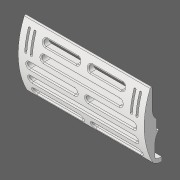
# Autodesk Inventor part: HandPlate
Saved by Autodesk Inventor 2020 (Build 240168000, 168)
## iProperties
Created: 2020-01-12
Part Number: HandPlate
Material: PLA Plastic (Black)
Document SubType Name: Modeling
Designer: Isaac Newcomb
Density: 1 g/cm^3
Appearance: 3D Printed - Black
Mass: 87.7555 g
Surface Area: 405.858 cm^2
Volume: 87.7555 cm^3
Author: Isaac Newcomb
Autodesk Inventor part; units mm, degrees
ref_plane "YZ Plane" through (0, 0, 0) normal (1, 0, 0) x (0, 1, 0)
ref_plane "XZ Plane" through (0, 0, 0) normal (0, 1, 0) x (-1, 0, 0)
ref_plane "XY Plane" through (0, 0, 0) normal (0, 0, 1) x (1, 0, 0)
sketch "Profile" plane through (0, 0, 0) normal (0, 0, 1) x (1, 0, 0)
  arc A0 (-13.7625, 56.5) -> (-16.6445, 57.0832) centre (-15.2625, 56.5) ccw
  line L0 (-7.7625, 0) -> (-7.7625, 15)
  arc A1 (-13.7625, 29.2829) -> (-7.7625, 15) centre (6.2375, 29.2829) ccw
  arc A2 (-16.6445, 57.0832) -> (-12.8608, -36.4892) centre (84.7024, 14.3185) ccw
  line L1 (0, 0) -> (-7.7625, 0)
  line L2 (-13.7625, 56.5) -> (-13.7625, 29.2829)
  line L3 (0, -41.5035) -> (0, -35.5035)
  line L4 (0, -35.5035) -> (-7.7625, -35.5035) construction
  arc A3 (-12.8608, -36.4892) -> (-12, -37.5035) centre (-10.2, -35.1035) ccw
  arc A4 (-9.8812, -31.3441) -> (-7.8643, -34.1785) centre (-6.8812, -31.3441) ccw
  arc A5 (-12, -37.5035) -> (0, -41.5035) centre (0, -21.5035) ccw
  line L5 (0, -41.5035) -> (-7.7625, -41.5035) construction
  arc A6 (-7.8643, -34.1785) -> (0, -35.5035) centre (0, -11.5035) ccw
  line L6 (-9.8812, -14.2829) -> (-9.8812, -31.3441)
  arc A7 (-3.8812, 0) -> (-9.8812, -14.2829) centre (10.1188, -14.2829) ccw
  dimension "height" = 56.5
  dimension "d3" = 1.5
  dimension "d5" = 15
  dimension "d100" = 110
  dimension "d114" = 20
  dimension "d115" = 7.7625
  dimension "d122" = 6
  dimension "d124" = 6
  dimension "d127" = 3
  dimension "d129" = 20
  dimension "d130" = 41.5035
  dimension "d131" = 12
  dimension "d133" = 20
  dimension "d134" = 6
  dimension "d135" = 3
  dimension "d136" = 10
  constraints: 17 point on circle, 14 end point, 10 tangent, 8 centre point, 4 vertical, 3 point on line, 2 midpoint, 2 perpendicular, 1 horizontal
  measures "height" vertical distance of A0.centre L1.start
  measures "d3" radius of A0
  measures "d5" distance of L0.start L0.end
  measures "d100" radius of A2
  measures "d114" radius of A1
  measures "d115" distance from line of L0 L1.start
  measures "d122" distance from line of L0 L2.start
  measures "d124" distance of L3.start L3.end
  measures "d127" radius of A3
  measures "d129" radius of A5
  measures "d130" distance of L1.start L3.start
  measures "d131" horizontal distance of L3.start A3.end
  measures "d133" radius of A7
  measures "d134" distance from line of A7.start L6
  measures "d135" radius of A4
  measures "d136" distance of A6.centre A5.centre
extrude "Extrusion" add sketch "Profile" along normal blind 180
sketch "Slot Sketch" plane through (0, 0, 0) normal (0, 1, 0) x (-1, 0, 0)
  line L0 (7.7625, 7.5) -> (10.7625, 9) construction
  line L1 (10.7625, 9) -> (10.7625, 3) construction
  line L2 (10.7625, 3) -> (7.7625, 4.5) construction
  line L3 (7.7625, 4.5) -> (7.7625, 7.5)
  line L4 (7.7625, 6) -> (11.2625, 6) construction
  line L5 (7.7625, 4.5) -> (7.7625, 3.941)
  line L6 (7.7625, 3.941) -> (11.2625, 2.191)
  line L7 (11.2625, 2.191) -> (11.2625, 9.809)
  line L8 (11.2625, 9.809) -> (7.7625, 8.059)
  line L9 (7.7625, 8.059) -> (7.7625, 7.5)
  line L10 (7.7625, 175.5) -> (10.7625, 177) construction
  line L11 (10.7625, 177) -> (10.7625, 171) construction
  line L12 (10.7625, 171) -> (7.7625, 172.5) construction
  line L13 (7.7625, 172.5) -> (7.7625, 175.5)
  line L14 (7.7625, 174) -> (11.2625, 174) construction
  line L15 (7.7625, 172.5) -> (7.7625, 171.941)
  line L16 (7.7625, 171.941) -> (11.2625, 170.191)
  line L17 (11.2625, 170.191) -> (11.2625, 177.809)
  line L18 (11.2625, 177.809) -> (7.7625, 176.059)
  line L19 (7.7625, 176.059) -> (7.7625, 175.5)
  line L20 (7.7625, 91.5) -> (10.7625, 93) construction
  line L21 (10.7625, 93) -> (10.7625, 87) construction
  line L22 (10.7625, 87) -> (7.7625, 88.5) construction
  line L23 (7.7625, 88.5) -> (7.7625, 91.5)
  line L24 (7.7625, 90) -> (11.2625, 90) construction
  line L25 (7.7625, 88.5) -> (7.7625, 87.941)
  line L26 (7.7625, 87.941) -> (11.2625, 86.191)
  line L27 (11.2625, 86.191) -> (11.2625, 93.809)
  line L28 (11.2625, 93.809) -> (7.7625, 92.059)
  line L29 (7.7625, 92.059) -> (7.7625, 91.5)
  point P0 (0, 0)
  point P1 (10.7625, 6)
  point P2 (10.7625, 174)
  point P3 (10.7625, 90)
  dimension "d14" = 0.5
  dimension "d15" = 0.5
  dimension "d16" = 3
  dimension "d17" = 6
  dimension "d18" = 3
  dimension "d19" = 7.7625
  dimension "d20" = 6
  dimension "d26" = 0.5
  dimension "d27" = 0.5
  dimension "d28" = 3
  dimension "d29" = 6
  dimension "d30" = 3
  dimension "d35" = 168
  dimension "d36" = 0.5
  dimension "d37" = 0.5
  dimension "d38" = 3
  dimension "d39" = 6
  dimension "d40" = 3
  dimension "d45" = 84
  constraints: 60 end point, 9 midpoint, 9 vertical, 6 parallel, 6 point on line, 5 collinear, 3 horizontal
  measures "d14" distance between parallel lines of L7 L1
  measures "d15" distance between parallel lines of L0 L8
  measures "d16" distance between parallel lines of L3 L1
  measures "d17" distance of L0.end L1.end
  measures "d18" distance of L2.end L0.start
  measures "d19" distance from line of point (0, 0) L3
  measures "d20" distance from line of point (0, 0) L4
  measures "d26" distance between parallel lines of L17 L11
  measures "d27" distance between parallel lines of L10 L18
  measures "d28" distance between parallel lines of L13 L11
  measures "d29" distance of L10.end L11.end
  measures "d30" distance of L12.end L10.start
  measures "d35" distance between parallel lines of L14 L4
  measures "d36" distance between parallel lines of L27 L21
  measures "d37" distance between parallel lines of L20 L28
  measures "d38" distance between parallel lines of L23 L21
  measures "d39" distance of L20.end L22.start
  measures "d40" distance of L22.end L23.end
  measures "d45" distance between parallel lines of L4 L24
extrude "Slots" cut sketch "Slot Sketch" along normal through all
sketch "Sketch3" plane through (0, 0, 0) normal (1, 0, 0) x (0, 1, 0)
  line L0 (50, 171) -> (20, 171)
  line L1 (20, 171) -> (20, 168)
  line L2 (20, 168) -> (50, 168)
  line L3 (50, 168) -> (50, 171)
  line L4 (50, 12) -> (20, 12)
  line L5 (20, 12) -> (20, 9)
  line L6 (20, 9) -> (50, 9)
  line L7 (50, 9) -> (50, 12)
  line L8 (35, 12) -> (35, 168) construction
  line L9 (20, 20) -> (50, 20)
  line L10 (50, 20) -> (50, 17)
  line L11 (50, 17) -> (20, 17)
  line L12 (20, 17) -> (20, 20)
  line L13 (20, 163) -> (50, 163)
  line L14 (50, 163) -> (50, 160)
  line L15 (50, 160) -> (20, 160)
  line L16 (20, 160) -> (20, 163)
  point P0 (0, 0)
  point P1 (35, 90)
  dimension "d48" = 90
  dimension "d50" = 20
  dimension "d51" = 30
  dimension "d52" = 3
  dimension "d53" = 12
  dimension "d56" = 5
  dimension "d57" = 5
  constraints: 34 end point, 8 parallel, 5 collinear, 4 horizontal, 4 perpendicular, 4 point on line, 3 midpoint
  measures "d48" vertical distance of point (0, 0) point (35, 90)
  measures "d50" distance from line of L5 point (0, 0)
  measures "d51" distance of L5.end L6.end
  measures "d52" distance of L6.end L4.start
  measures "d53" distance from line of point (0, 0) L4
  measures "d56" distance between parallel lines of L2 L13
  measures "d57" distance between parallel lines of L4 L11
extrude "Extrusion3" cut sketch "Sketch3" against normal through all
fillet "Fillet2" radius 1.5 16 edges at (-16.5561, 50, 12) (-18.3143, 20, 12) (-18.3143, 20, 9) (-16.5561, 50, 9) (-16.5561, 50, 163) (-18.3143, 20, 163) (-18.3143, 20, 160) (-16.5561, 50, 160) (-18.3143, 20, 168) (-16.5561, 50, 168) (-18.3143, 20, 171) (-16.5561, 50, 171) (-16.5561, 50, 20) (-16.5561, 50, 17) (-18.3143, 20, 17) (-18.3143, 20, 20)
sketch "Sketch4" plane through (0, 0, 0) normal (1, 0, 0) x (0, 1, 0)
  line L0 (25.5, 144) -> (25.5, 36) construction
  line L1 (21.5, 144) -> (21.5, 36)
  line L2 (29.5, 36) -> (29.5, 144)
  arc A0 (29.5, 144) -> (21.5, 144) centre (25.5, 144) ccw
  arc A1 (21.5, 36) -> (29.5, 36) centre (25.5, 36) ccw
  line L3 (25.5, 90) -> (21.5, 90) construction
  line L4 (-10.5, 164) -> (-10.5, 16) construction
  line L5 (-14.5, 164) -> (-14.5, 16)
  line L6 (-6.5, 16) -> (-6.5, 164)
  arc A2 (-6.5, 164) -> (-14.5, 164) centre (-10.5, 164) ccw
  arc A3 (-14.5, 16) -> (-6.5, 16) centre (-10.5, 16) ccw
  line L7 (7.5, 164) -> (7.5, 100) construction
  line L8 (3.5, 164) -> (3.5, 100)
  line L9 (11.5, 100) -> (11.5, 164)
  arc A4 (11.5, 164) -> (3.5, 164) centre (7.5, 164) ccw
  arc A5 (3.5, 100) -> (11.5, 100) centre (7.5, 100) ccw
  line L10 (7.5, 80) -> (7.5, 16) construction
  line L11 (3.5, 80) -> (3.5, 16)
  line L12 (11.5, 16) -> (11.5, 80)
  arc A6 (11.5, 80) -> (3.5, 80) centre (7.5, 80) ccw
  arc A7 (3.5, 16) -> (11.5, 16) centre (7.5, 16) ccw
  line L13 (7.5, 80) -> (7.5, 100) construction
  line L14 (-28.5, 80) -> (-28.5, 16) construction
  line L15 (-32.5, 80) -> (-32.5, 16)
  line L16 (-24.5, 16) -> (-24.5, 80)
  arc A8 (-24.5, 80) -> (-32.5, 80) centre (-28.5, 80) ccw
  arc A9 (-32.5, 16) -> (-24.5, 16) centre (-28.5, 16) ccw
  line L17 (-28.5, 164) -> (-28.5, 100) construction
  line L18 (-32.5, 164) -> (-32.5, 100)
  line L19 (-24.5, 100) -> (-24.5, 164)
  arc A10 (-24.5, 164) -> (-32.5, 164) centre (-28.5, 164) ccw
  arc A11 (-32.5, 100) -> (-24.5, 100) centre (-28.5, 100) ccw
  line L20 (-28.5, 100) -> (-28.5, 80) construction
  line L21 (43.5, 144) -> (43.5, 100) construction
  line L22 (39.5, 144) -> (39.5, 100)
  line L23 (47.5, 100) -> (47.5, 144)
  arc A12 (47.5, 144) -> (39.5, 144) centre (43.5, 144) ccw
  arc A13 (39.5, 100) -> (47.5, 100) centre (43.5, 100) ccw
  line L24 (43.5, 80) -> (43.5, 36) construction
  line L25 (39.5, 80) -> (39.5, 36)
  line L26 (47.5, 36) -> (47.5, 80)
  arc A14 (47.5, 80) -> (39.5, 80) centre (43.5, 80) ccw
  arc A15 (39.5, 36) -> (47.5, 36) centre (43.5, 36) ccw
  line L27 (43.5, 80) -> (43.5, 100) construction
  point P0 (0, 0)
  point P1 (-10.5, 90)
  point P2 (7.5, 132)
  point P3 (7.5, 48)
  point P4 (7.5, 90)
  point P5 (-28.5, 48)
  point P6 (-28.5, 132)
  point P7 (-28.5, 90)
  point P8 (43.5, 122)
  point P9 (43.5, 58)
  point P10 (43.5, 90)
  dimension "d59" = 4
  dimension "d62" = 108
  dimension "d83" = 90
  dimension "d85" = 7.5
  dimension "d86" = 16
  dimension "d87" = 10
  dimension "d88" = 10
  dimension "d89" = 10
  dimension "d92" = 16
  dimension "d95" = 10
  dimension "d96" = 16
  dimension "d97" = 10
  dimension "d98" = 108
  dimension "d99" = 10
  constraints: 72 end point, 32 point on circle, 32 tangent, 16 centre point, 12 midpoint, 10 point on line, 8 parallel, 8 vertical, 7 equal radius, 4 equal length, 1 horizontal
  measures "d59" radius of A1
  measures "d62" distance of L0.start L0.end
  measures "d83" distance from line of point (0, 0) L3
  measures "d85" distance from line of point (0, 0) L10
  measures "d86" vertical distance of point (0, 0) L10.end
  measures "d87" distance of point (7.5, 90) L10.start
  measures "d88" distance between parallel lines of L8 L6
  measures "d89" distance between parallel lines of L1 L9
  measures "d92" vertical distance of L4.end point (0, 0)
  measures "d95" distance between parallel lines of L5 L19
  measures "d96" vertical distance of L14.end point (0, 0)
  measures "d97" distance of L24.start point (43.5, 90)
  measures "d98" distance of L21.start L24.end
  measures "d99" distance between parallel lines of L2 L22
extrude "Extrusion4" cut sketch "Sketch4" against normal through all
fillet "Fillet3" radius 1.5 32 edges at (-21.3501, 43.5225, 32.0001) (-20.1737, 47.5, 58) (-21.3539, 43.5086, 84) (-22.3766, 39.5, 58) (-20.1737, 47.5, 122) (-21.3539, 43.5086, 148) (-22.3766, 39.5, 122) (-21.3501, 43.5225, 96.0001) (-24.7318, 25.4613, 147.9998) (-25.063, 21.5, 90) (-24.7275, 25.5033, 32) (-24.245, 29.5, 90) (-25.2615, 11.5, 132) (-25.0823, 7.4398, 167.9995) (-24.7643, 3.5, 132) (-25.0855, 7.4896, 96) (-25.0855, 7.4896, 12) (-25.2615, 11.5, 48) (-25.0823, 7.4398, 83.9995) (-24.7643, 3.5, 48) (-22.4558, -10.5234, 12.0001) (-23.3096, -6.5, 90) (-22.4577, -10.5153, 168) (-21.4555, -14.5, 90) (-16.6051, -28.5394, 12.0002) (-18.2205, -24.5, 48) (-16.6104, -28.5268, 83.9999) (-14.8367, -32.5, 48) (-16.6104, -28.5268, 167.9999) (-14.8367, -32.5, 132) (-16.6051, -28.5394, 96.0002) (-18.2205, -24.5, 132)
equation "\"d14\" = tabTol"
equation "\"d15\" = tabTol"
equation "\"d16\" = bigTabHeight"
equation "\"d17\" = bigTabTopWidth"
equation "\"d18\" = bigTabBaseWidth"
equation "\"d5\" = boxWidth"
equation "\"d0\" = 15 * chanWidth"
equation "\"d19\" = boxHeight"
equation "\"tabTol\" = 0.5"
equation "\"d31\" = 0.2"
equation "\"d41\" = 0.2"
equation "\"bigTabHeight\" = 3"
equation "\"bigTabTopWidth\" = 6"
equation "\"bigTabBaseWidth\" = 3"
equation "\"boxWidth\" = 15"
equation "\"chanWidth\" = 12"
equation "\"boxHeight\" = 7.7625"
body "Solid1"
